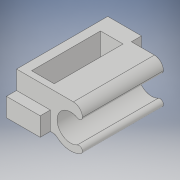
# Autodesk Inventor part: Switch holder_Right
Saved by Autodesk Inventor 2019 (Build 230136000, 136)
## iProperties
Created: 2019-09-19
Part Number: Switch holder_Right
Material: Generic
Document SubType Name: Modeling
Designer: 19879326
Density: 1 g/cm^3
Appearance: Default
Author: 19879326
Autodesk Inventor part; units mm, degrees
ref_plane "YZ Plane" through (0, 0, 0) normal (1, 0, 0) x (0, 1, 0)
ref_plane "XZ Plane" through (0, 0, 0) normal (0, 1, 0) x (-1, 0, 0)
ref_plane "XY Plane" through (0, 0, 0) normal (0, 0, 1) x (1, 0, 0)
sketch "Sketch1" plane through (0, 0, 0) normal (0, 0, 1) x (1, 0, 0)
  line L0 (-6, 5.5) -> (6, 5.5)
  line L1 (6, 5.5) -> (6, -5.5)
  line L2 (6, -5.5) -> (-6, -5.5)
  line L3 (-6, -5.5) -> (-6, 5.5)
  point P0 (0, 0)
  point P1 (6, 0)
  point P2 (0, 5.5)
  dimension "d0" = 12
  dimension "d1" = 11
  constraints: 8 end point, 2 midpoint, 2 parallel, 1 horizontal, 1 horizontal alignment, 1 perpendicular, 1 vertical alignment
  measures "d0" distance of L0.start L0.end
  measures "d1" distance of L0.end L1.end
extrude "Extrusion1" add sketch "Sketch1" along normal blind 24
sketch "Sketch2" plane through (-6, 5.5, 0) normal (0, 1, 0) x (1, 0, 0)
  line L0 (2.65, -22.2) -> (9.35, -22.2)
  line L1 (9.35, -22.2) -> (9.35, -1.8)
  line L2 (9.35, -1.8) -> (2.65, -1.8)
  line L3 (2.65, -1.8) -> (2.65, -22.2)
  line L4 (0, 0) -> (0, -24) projected
  line L5 (0, 0) -> (12, 0) projected
  point P0 (6, 0)
  point P1 (2.65, -12)
  point P2 (0, -12)
  point P3 (6, -1.8)
  point P4 (6, 0)
  dimension "d4" = 20.4
  dimension "d5" = 6.7
  constraints: 8 end point, 4 midpoint, 2 parallel, 1 horizontal, 1 horizontal alignment, 1 perpendicular, 1 vertical alignment
  measures "d4" distance of L2.end L0.start
  measures "d5" distance of L1.end L2.end
extrude "Extrusion2" cut sketch "Sketch2" against normal blind 10
sketch "Sketch3" plane through (-6, -4.5, 0) normal (0, 1, 0) x (1, 0, 0)
  line L0 (2.65, -22.2) -> (2.65, -1.8) projected
  line L1 (9.35, -1.8) -> (9.35, -22.2) projected
  line L2 (2.65, -21.5) -> (9.35, -21.5)
  line L3 (9.35, -21.5) -> (9.35, -18.3)
  line L4 (9.35, -18.3) -> (2.65, -18.3)
  line L5 (2.65, -18.3) -> (2.65, -21.5)
  line L6 (2.65, -14.2) -> (9.35, -14.2)
  line L7 (9.35, -14.2) -> (9.35, -11)
  line L8 (9.35, -11) -> (2.65, -11)
  line L9 (2.65, -11) -> (2.65, -14.2)
  line L10 (2.65, -5.4) -> (9.35, -5.4)
  line L11 (9.35, -5.4) -> (9.35, -2.2)
  line L12 (9.35, -2.2) -> (2.65, -2.2)
  line L13 (2.65, -2.2) -> (2.65, -5.4)
  line L14 (9.35, -22.2) -> (2.65, -22.2) projected
  line L15 (2.65, -1.8) -> (9.35, -1.8) projected
  point P0 (6, 0)
  point P1 (2.65, -19.9)
  point P2 (2.65, -12.6)
  point P3 (2.65, -3.8)
  dimension "d9" = 7.3
  dimension "d10" = 8.8
  dimension "d11" = 3.2
  dimension "d12" = 3.2
  dimension "d13" = 3.2
  dimension "d39" = 2
  constraints: 24 end point, 6 parallel, 6 point on line, 3 horizontal, 3 midpoint, 3 perpendicular
  measures "d9" distance of point (2.65, -12.6) point (2.65, -19.9)
  measures "d10" distance of point (2.65, -3.8) point (2.65, -12.6)
  measures "d11" distance between parallel lines of L4 L2
  measures "d12" distance of L8.end L6.start
  measures "d13" distance between parallel lines of L10 L12
  measures "d39" distance from line of L15 point (2.65, -3.8)
extrude "Extrusion3" cut sketch "Sketch3" against normal blind 10 contours L0 L4 L1 L2 | L0 L8 L1 L6 | L0 L12 L1 L10
sketch "Sketch4" plane through (0, 0, 24) normal (0, 0, 1) x (1, 0, 0)
  line L0 (6, 5.5) -> (-6, 5.5) projected
  circle A0 centre (10, -1.5) radius 4
  arc A1 (6, 2.9721) -> (13, -6.6962) centre (10, -1.5) ccw
  arc A2 (12, 1.9641) -> (13.5, 2.8301) centre (12.5, 2.8301) ccw
  arc A3 (13, -6.6962) -> (12, -4.9641) centre (12.5, -5.8301) ccw
  line L1 (6, -5.5) -> (6, 5.5) projected
  line L2 (6, 2.9721) -> (6, -5.9721)
  circle A4 centre (10, -1.5) radius 4
  arc A5 (6, 2.9721) -> (13, -6.6962) centre (10, -1.5) ccw
  line L3 (6, 5.5) -> (10.8301, 5.5)
  line L4 (6, 5.5) -> (6, 2.9721)
  arc A6 (13.5, 2.8301) -> (10.8301, 5.5) centre (10.8301, 2.8301) ccw
  point P0 (0, 0)
  dimension "d31" = 8
  dimension "d32" = 12
  dimension "d33" = 7
  dimension "d34" = 2.5
  constraints: 13 point on circle, 7 centre point, 7 tangent, 6 end point, 3 coincident, 2 concentric, 2 point on line, 1 horizontal, 1 horizontal alignment, 1 perpendicular, 1 vertical alignment
  measures "d31" diameter of A0
  measures "d32" diameter of A1
  measures "d33" distance from line of L0 A0.centre
  measures "d34" horizontal distance of A0.centre A2.centre
extrude "Extrusion4" add sketch "Sketch4" against normal blind 24 contours A0 L1 L3 A6 A2 | A3 A1 L2 L1 A0 | L1 L2 A1
sketch "Sketch5" plane through (0, 0, 0) normal (0, 0, -1) x (-1, 0, 0)
  line L0 (6, 5.5) -> (-6, 5.5) projected
  line L1 (6, 5.5) -> (-4, 5.5)
  line L2 (-4, 5.5) -> (-4, 0)
  line L3 (-4, 0) -> (6, 0)
  line L4 (6, 0) -> (6, 5.5)
  dimension "d35" = 10
  dimension "d36" = 5.5
  constraints: 8 end point, 2 parallel, 1 horizontal, 1 perpendicular
  measures "d35" distance of L3.end L2.end
  measures "d36" distance of L2.end L1.end
extrude "Extrusion5" add sketch "Sketch5" along normal blind 3
sketch "Sketch6" plane through (0, 0, 24) normal (0, 0, 1) x (1, 0, 0)
  line L0 (-6, -5.5) -> (-6, 0) projected
  line L1 (-6, -5.5) -> (4, -5.5)
  line L2 (4, -5.5) -> (4, 0)
  line L3 (4, 0) -> (-6, 0)
  line L4 (-6, 0) -> (-6, -5.5)
  dimension "d37" = 10
  dimension "d38" = 5.5
  constraints: 8 end point, 2 parallel, 1 horizontal, 1 perpendicular
  measures "d37" distance of L3.end L2.end
  measures "d38" distance of L2.end L1.end
extrude "Extrusion6" add sketch "Sketch6" along normal blind 3
fillet "Fillet2" radius 2 1 edges at (5.5279, -5.5, 12)
body "Solid1"
